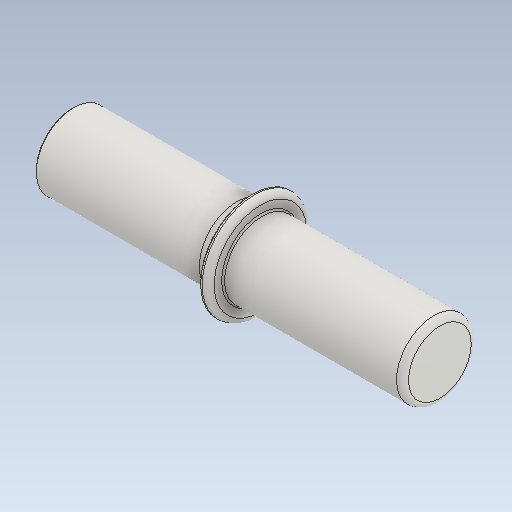
# Autodesk Inventor part: Shaft
Saved by Autodesk Inventor 2021 (Build 250183000, 183)
## iProperties
Created: 2023-06-22
Part Number: Shaft
Material: Steel
Document SubType Name: Modeling
Designer: mahmo
Density: 1 g/cm^3
Appearance: Steel
CustomPartVersion: 1
Author: mahmo
Length: 123.000 mm
Autodesk Inventor part; units mm, degrees
ref_plane "Start Plane" through (0, 0, 0) normal (1, 0, 0) x (0, 1, 0)
ref_plane "XZ Plane" through (0, 0, 0) normal (0, 1, 0) x (-1, 0, 0)
ref_plane "XY Plane" through (0, 0, 0) normal (0, 0, 1) x (1, 0, 0)
sketch "Main Sketch" plane through (0, 0, 0) normal (0, 0, 1) x (1, 0, 0)
  line L0 (0, 0) -> (123, 0)
  line L1 (0, 0) -> (0, 12.5)
  line L2 (0, 12.5) -> (60, 12.5)
  line L3 (60, 12.5) -> (60, 17.5)
  line L4 (63, 17.5) -> (63, 12.5)
  line L5 (60, 17.5) -> (63, 17.5)
  line L6 (123, 12.5) -> (123, 0)
  line L7 (63, 12.5) -> (123, 12.5)
  dimension "d3" = 25
  dimension "d4" = 35
  dimension "d5" = 25
  constraints: 16 end point, 5 horizontal, 4 vertical
  measures "d3" diameter of L2 L0
  measures "d4" diameter of L5 L0
  measures "d5" diameter of L7 L0
revolve "Revolution1" add sketch "Main Sketch" angle 360 about axis through (0, 0, 0) along (1, 0, 0)
chamfer "Chamfer3" distance 0.5 angle 45 1 edges at (60, -17.5, 0) measured on face at (62, 17.4433, -1.4082)
fillet "Fillet2" radius 2 1 edges at (63, -17.5, 0)
chamfer "Chamfer4" distance 0.5 angle 45 1 edges at (63, -12.5, 0) measured on face at (103, 12.4595, -1.0058)
fillet "Fillet3" radius 2 1 edges at (123, -12.5, 0)
chamfer "Chamfer1" distance 0.5 angle 45 1 edges at (0, -12.5, 0) measured on face at (40, 12.4595, -1.0058)
fillet "Fillet1" radius 5 1 edges at (60, -12.5, 0)
equation "\"Length\" = 123"
body "Solid1"
